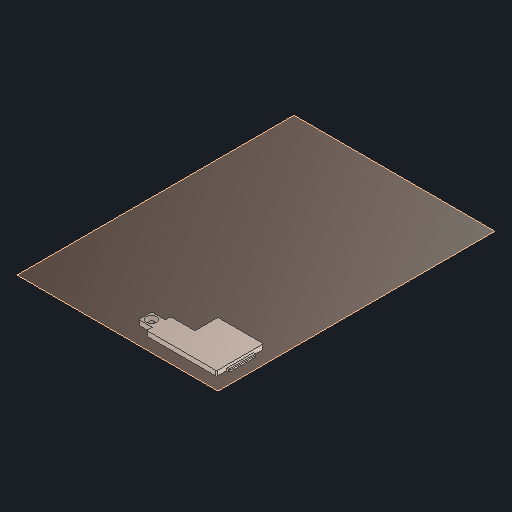
# Autodesk Inventor part: Kameraturm_Abdeckung_Unten
Saved by Autodesk Inventor 2026.1 (Build 301233020, 233B)
## iProperties
Created: 2025-10-16
Part Number: Kameraturm_Abdeckung_Unten
Material: Generisch
Document SubType Name: Modeling
Designer: iopeter
Density: 1 g/cm^3
Appearance: Vorgabe
Author: iopeter
Autodesk Inventor part; units mm, degrees
ref_plane "YZ Plane" through (0, 0, 0) normal (1, 0, 0) x (0, 1, 0)
ref_plane "XZ Plane" through (0, 0, 0) normal (0, 1, 0) x (-1, 0, 0)
ref_plane "XY Plane" through (0, 0, 0) normal (0, 0, 1) x (1, 0, 0)
ref_plane "Arbeitsebene1" through (-7.5, 0, 0) normal (0, 0, 1) x (1, 0, 0)
sketch "Skizze1" plane through (-7.5, 0, 0) normal (0, 0, 1) x (1, 0, 0)
  line L0 (-71.1, -93.5) -> (-71.1, 90.5) projected
  line L1 (62.9, -94.5) -> (-70.1, -94.5) projected
  line L2 (63.9, 90.5) -> (63.9, -93.5) projected
  line L3 (-70.1, 91.5) -> (62.9, 91.5) projected
  line L4 (23.9, -70.5) -> (-66.1, -70.5) projected
  line L5 (-66.1, -70.5) -> (-66.1, 73.5) projected
  line L6 (-66.1, 73.5) -> (23.9, 73.5) projected
  line L7 (23.9, 73.5) -> (23.9, -70.5) projected
  line L8 (8.9, -87.5) -> (-1.1, -87.5) projected
  line L9 (-1.1, -87.5) -> (-1.1, -77.5) projected
  line L10 (-1.1, -77.5) -> (8.9, -77.5) projected
  line L11 (8.9, -77.5) -> (8.9, -73.5) projected
  line L12 (8.9, -73.5) -> (26.9, -73.5) projected
  line L13 (26.9, -73.5) -> (26.9, -56.5) projected
  line L14 (26.9, -56.5) -> (60.9, -56.5) projected
  line L15 (60.9, -56.5) -> (60.9, -91.5) projected
  line L16 (60.9, -91.5) -> (8.9, -91.5) projected
  line L17 (8.9, -91.5) -> (8.9, -87.5) projected
  line L18 (-0.95, -77.65) -> (-0.95, -87.35)
  line L19 (-0.95, -87.35) -> (9.05, -87.35)
  line L20 (9.05, -87.35) -> (9.05, -91.35)
  line L21 (9.05, -91.35) -> (60.75, -91.35)
  line L22 (60.75, -91.35) -> (60.75, -56.65)
  line L23 (60.75, -56.65) -> (27.05, -56.65)
  line L24 (27.05, -56.65) -> (27.05, -73.65)
  line L25 (27.05, -73.65) -> (9.05, -73.65)
  line L26 (9.05, -73.65) -> (9.05, -77.65)
  line L27 (9.05, -77.65) -> (-0.95, -77.65)
  line L28 (63.9, -93.5) -> (62.9, -94.5) projected
  line L29 (62.9, 91.5) -> (63.9, 90.5) projected
  line L30 (-71.1, 90.5) -> (-70.1, 91.5) projected
  line L31 (-70.1, -94.5) -> (-71.1, -93.5) projected
  circle A0 centre (43.9, -1.5) radius 7.55 projected
  circle A1 centre (-61.1, -85.5) radius 7.55 projected
  circle A2 centre (-61.1, 82.5) radius 7.55 projected
  point P0 (7.5, 0)
  dimension "d0" = 0.15
  constraints: 20 end point, 9 other
  measures "d0" distance between parallel lines of L9 L18
extrude "Extrusion1" add sketch "Skizze1" against normal blind 3.6 contours L27 L26 L25 L24 L23 L22 L21 L20 L19 L18
sketch "Skizze2" plane through (-7.5, 0, 0) normal (0, 0, 1) x (1, 0, 0)
  circle A0 centre (3.9, -82.5) radius 2 projected
  point P0 (7.5, 0)
hole "Bohrung1" at (-3.6, -82.5, 0) direction (0, 0, -1) diameter 3.4 depth 8 countersink diameter 7.5 countersink angle 90 clearance for "Innensechskant-Senkkopfschraube DIN EN ISO 10642" size "M3" standard "DIN"
sketch "Skizze3" plane through (53.25, -91.35, 0) normal (1, 0, 0) x (0, 0, -1)
  line L0 (2, 27.35) -> (2, 7.35) projected
  line L1 (2, 7.35) -> (3.6, 7.35)
  line L2 (3.6, 7.35) -> (3.6, 27.35)
  line L3 (3.6, 27.35) -> (2, 27.35)
  line L4 (2, 27.35) -> (2, 7.35)
  point P0 (0, 91.35)
  point P1 (3.6, 34.7)
  constraints: 8 end point, 2 parallel, 1 horizontal, 1 horizontal alignment, 1 perpendicular, 1 vertical alignment
extrude "Extrusion2" add sketch "Skizze3" along normal blind 2
chamfer "Fasen1" distance 0.5 angle 45 7 edges at (-8.45, -87.35, -1.8) (-8.45, -77.65, -1.8) (1.55, -73.65, -1.8) (1.55, -91.35, -1.8) (19.55, -56.65, -1.8) (53.25, -56.65, -1.8) (53.25, -91.35, -1.8)
chamfer "Fasen2" distance 0.5 angle 45 3 edges at (55.25, -84, -2.8) (55.25, -64, -2.8) (55.25, -74, -2)
